Autodesk Inventor part; units mm, degrees
(part 2 of 2)
  line L623 (86.4105, 126.8852) -> (86.4105, 127.8852)
  line L624 (86.4105, 127.8852) -> (84.4105, 127.8852)
  line L625 (84.4105, 127.8852) -> (84.4105, 125.8852)
  line L626 (84.4105, 125.8852) -> (86.4105, 125.8852)
  line L627 (86.4105, 127.8852) -> (86.4105, 125.8852)
  line L628 (86.4105, 136.8852) -> (86.4105, 137.8852)
  line L629 (86.4105, 137.8852) -> (84.4105, 137.8852)
  line L630 (84.4105, 137.8852) -> (84.4105, 135.8852)
  line L631 (84.4105, 135.8852) -> (86.4105, 135.8852)
  line L632 (86.4105, 137.8852) -> (86.4105, 135.8852)
  line L633 (86.4105, 146.8852) -> (86.4105, 147.8852)
  line L634 (86.4105, 147.8852) -> (84.4105, 147.8852)
  line L635 (84.4105, 147.8852) -> (84.4105, 145.8852)
  line L636 (84.4105, 145.8852) -> (86.4105, 145.8852)
  line L637 (86.4105, 147.8852) -> (86.4105, 145.8852)
  line L638 (86.4105, 156.8852) -> (86.4105, 157.8852)
  line L639 (86.4105, 157.8852) -> (84.4105, 157.8852)
  line L640 (84.4105, 157.8852) -> (84.4105, 155.8852)
  line L641 (84.4105, 155.8852) -> (86.4105, 155.8852)
  line L642 (86.4105, 157.8852) -> (86.4105, 155.8852)
  line L643 (86.4105, 166.8852) -> (86.4105, 167.8852)
  line L644 (86.4105, 167.8852) -> (84.4105, 167.8852)
  line L645 (84.4105, 167.8852) -> (84.4105, 165.8852)
  line L646 (84.4105, 165.8852) -> (86.4105, 165.8852)
  line L647 (86.4105, 167.8852) -> (86.4105, 165.8852)
  line L648 (86.4105, 176.8852) -> (86.4105, 177.8852)
  line L649 (86.4105, 177.8852) -> (84.4105, 177.8852)
  line L650 (84.4105, 177.8852) -> (84.4105, 175.8852)
  line L651 (84.4105, 175.8852) -> (86.4105, 175.8852)
  line L652 (86.4105, 177.8852) -> (86.4105, 175.8852)
  line L653 (86.4105, 46.8852) -> (86.4105, 47.8852)
  line L654 (86.4105, 47.8852) -> (84.4105, 47.8852)
  line L655 (84.4105, 47.8852) -> (84.4105, 45.8852)
  line L656 (84.4105, 45.8852) -> (86.4105, 45.8852)
  line L657 (86.4105, 47.8852) -> (86.4105, 45.8852)
  line L658 (86.4105, 56.8852) -> (86.4105, 57.8852)
  line L659 (86.4105, 57.8852) -> (84.4105, 57.8852)
  line L660 (84.4105, 57.8852) -> (84.4105, 55.8852)
  line L661 (84.4105, 55.8852) -> (86.4105, 55.8852)
  line L662 (86.4105, 57.8852) -> (86.4105, 55.8852)
  line L663 (86.4105, 66.8852) -> (86.4105, 67.8852)
  line L664 (86.4105, 67.8852) -> (84.4105, 67.8852)
  line L665 (84.4105, 67.8852) -> (84.4105, 65.8852)
  line L666 (84.4105, 65.8852) -> (86.4105, 65.8852)
  line L667 (86.4105, 67.8852) -> (86.4105, 65.8852)
  line L668 (86.4105, 76.8852) -> (86.4105, 77.8852)
  line L669 (86.4105, 77.8852) -> (84.4105, 77.8852)
  line L670 (84.4105, 77.8852) -> (84.4105, 75.8852)
  line L671 (84.4105, 75.8852) -> (86.4105, 75.8852)
  line L672 (86.4105, 77.8852) -> (86.4105, 75.8852)
  line L673 (86.4105, 86.8852) -> (86.4105, 87.8852)
  line L674 (86.4105, 87.8852) -> (84.4105, 87.8852)
  line L675 (84.4105, 87.8852) -> (84.4105, 85.8852)
  line L676 (84.4105, 85.8852) -> (86.4105, 85.8852)
  line L677 (86.4105, 87.8852) -> (86.4105, 85.8852)
  line L678 (86.4105, 96.8852) -> (86.4105, 97.8852)
  line L679 (86.4105, 97.8852) -> (84.4105, 97.8852)
  line L680 (84.4105, 97.8852) -> (84.4105, 95.8852)
  line L681 (84.4105, 95.8852) -> (86.4105, 95.8852)
  line L682 (86.4105, 97.8852) -> (86.4105, 95.8852)
  line L683 (86.4105, 106.8852) -> (86.4105, 107.8852)
  line L684 (86.4105, 107.8852) -> (84.4105, 107.8852)
  line L685 (84.4105, 107.8852) -> (84.4105, 105.8852)
  line L686 (84.4105, 105.8852) -> (86.4105, 105.8852)
  line L687 (86.4105, 107.8852) -> (86.4105, 105.8852)
  line L688 (86.4105, 116.8852) -> (86.4105, 117.8852)
  line L689 (86.4105, 117.8852) -> (84.4105, 117.8852)
  line L690 (84.4105, 117.8852) -> (84.4105, 115.8852)
  line L691 (84.4105, 115.8852) -> (86.4105, 115.8852)
  line L692 (86.4105, 117.8852) -> (86.4105, 115.8852)
  line L693 (86.4105, 126.8852) -> (86.4105, 127.8852)
  line L694 (86.4105, 127.8852) -> (84.4105, 127.8852)
  line L695 (84.4105, 127.8852) -> (84.4105, 125.8852)
  line L696 (84.4105, 125.8852) -> (86.4105, 125.8852)
  line L697 (86.4105, 127.8852) -> (86.4105, 125.8852)
  line L698 (86.4105, 136.8852) -> (86.4105, 137.8852)
  line L699 (86.4105, 137.8852) -> (84.4105, 137.8852)
  line L700 (84.4105, 137.8852) -> (84.4105, 135.8852)
  line L701 (84.4105, 135.8852) -> (86.4105, 135.8852)
  line L702 (86.4105, 137.8852) -> (86.4105, 135.8852)
  line L703 (86.4105, 146.8852) -> (86.4105, 147.8852)
  line L704 (86.4105, 147.8852) -> (84.4105, 147.8852)
  line L705 (84.4105, 147.8852) -> (84.4105, 145.8852)
  line L706 (84.4105, 145.8852) -> (86.4105, 145.8852)
  line L707 (86.4105, 147.8852) -> (86.4105, 145.8852)
  line L708 (86.4105, 156.8852) -> (86.4105, 157.8852)
  line L709 (86.4105, 157.8852) -> (84.4105, 157.8852)
  line L710 (84.4105, 157.8852) -> (84.4105, 155.8852)
  line L711 (84.4105, 155.8852) -> (86.4105, 155.8852)
  line L712 (86.4105, 157.8852) -> (86.4105, 155.8852)
  line L713 (86.4105, 166.8852) -> (86.4105, 167.8852)
  line L714 (86.4105, 167.8852) -> (84.4105, 167.8852)
  line L715 (84.4105, 167.8852) -> (84.4105, 165.8852)
  line L716 (84.4105, 165.8852) -> (86.4105, 165.8852)
  line L717 (86.4105, 167.8852) -> (86.4105, 165.8852)
  line L718 (86.4105, 36.8852) -> (86.4105, 37.8852)
  line L719 (86.4105, 37.8852) -> (84.4105, 37.8852)
  line L720 (84.4105, 37.8852) -> (84.4105, 35.8852)
  line L721 (84.4105, 35.8852) -> (86.4105, 35.8852)
  line L722 (86.4105, 37.8852) -> (86.4105, 35.8852)
  line L723 (86.4105, 46.8852) -> (86.4105, 47.8852)
  line L724 (86.4105, 47.8852) -> (84.4105, 47.8852)
  line L725 (84.4105, 47.8852) -> (84.4105, 45.8852)
  line L726 (84.4105, 45.8852) -> (86.4105, 45.8852)
  line L727 (86.4105, 47.8852) -> (86.4105, 45.8852)
  line L728 (86.4105, 56.8852) -> (86.4105, 57.8852)
  line L729 (86.4105, 57.8852) -> (84.4105, 57.8852)
  line L730 (84.4105, 57.8852) -> (84.4105, 55.8852)
  line L731 (84.4105, 55.8852) -> (86.4105, 55.8852)
  line L732 (86.4105, 57.8852) -> (86.4105, 55.8852)
  line L733 (86.4105, 66.8852) -> (86.4105, 67.8852)
  line L734 (86.4105, 67.8852) -> (84.4105, 67.8852)
  line L735 (84.4105, 67.8852) -> (84.4105, 65.8852)
  line L736 (84.4105, 65.8852) -> (86.4105, 65.8852)
  line L737 (86.4105, 67.8852) -> (86.4105, 65.8852)
  line L738 (86.4105, 76.8852) -> (86.4105, 77.8852)
  line L739 (86.4105, 77.8852) -> (84.4105, 77.8852)
  line L740 (84.4105, 77.8852) -> (84.4105, 75.8852)
  line L741 (84.4105, 75.8852) -> (86.4105, 75.8852)
  line L742 (86.4105, 77.8852) -> (86.4105, 75.8852)
  line L743 (86.4105, 86.8852) -> (86.4105, 87.8852)
  line L744 (86.4105, 87.8852) -> (84.4105, 87.8852)
  line L745 (84.4105, 87.8852) -> (84.4105, 85.8852)
  line L746 (84.4105, 85.8852) -> (86.4105, 85.8852)
  line L747 (86.4105, 87.8852) -> (86.4105, 85.8852)
  line L748 (86.4105, 96.8852) -> (86.4105, 97.8852)
  line L749 (86.4105, 97.8852) -> (84.4105, 97.8852)
  line L750 (84.4105, 97.8852) -> (84.4105, 95.8852)
  line L751 (84.4105, 95.8852) -> (86.4105, 95.8852)
  line L752 (86.4105, 97.8852) -> (86.4105, 95.8852)
  line L753 (86.4105, 106.8852) -> (86.4105, 107.8852)
  line L754 (86.4105, 107.8852) -> (84.4105, 107.8852)
  line L755 (84.4105, 107.8852) -> (84.4105, 105.8852)
  line L756 (84.4105, 105.8852) -> (86.4105, 105.8852)
  line L757 (86.4105, 107.8852) -> (86.4105, 105.8852)
  line L758 (86.4105, 116.8852) -> (86.4105, 117.8852)
  line L759 (86.4105, 117.8852) -> (84.4105, 117.8852)
  line L760 (84.4105, 117.8852) -> (84.4105, 115.8852)
  line L761 (84.4105, 115.8852) -> (86.4105, 115.8852)
  line L762 (86.4105, 117.8852) -> (86.4105, 115.8852)
  line L763 (86.4105, 126.8852) -> (86.4105, 127.8852)
  line L764 (86.4105, 127.8852) -> (84.4105, 127.8852)
  line L765 (84.4105, 127.8852) -> (84.4105, 125.8852)
  line L766 (84.4105, 125.8852) -> (86.4105, 125.8852)
  line L767 (86.4105, 127.8852) -> (86.4105, 125.8852)
  line L768 (86.4105, 136.8852) -> (86.4105, 137.8852)
  line L769 (86.4105, 137.8852) -> (84.4105, 137.8852)
  line L770 (84.4105, 137.8852) -> (84.4105, 135.8852)
  line L771 (84.4105, 135.8852) -> (86.4105, 135.8852)
  line L772 (86.4105, 137.8852) -> (86.4105, 135.8852)
  line L773 (86.4105, 146.8852) -> (86.4105, 147.8852)
  line L774 (86.4105, 147.8852) -> (84.4105, 147.8852)
  line L775 (84.4105, 147.8852) -> (84.4105, 145.8852)
  line L776 (84.4105, 145.8852) -> (86.4105, 145.8852)
  line L777 (86.4105, 147.8852) -> (86.4105, 145.8852)
  line L778 (86.4105, 156.8852) -> (86.4105, 157.8852)
  line L779 (86.4105, 157.8852) -> (84.4105, 157.8852)
  line L780 (84.4105, 157.8852) -> (84.4105, 155.8852)
  line L781 (84.4105, 155.8852) -> (86.4105, 155.8852)
  line L782 (86.4105, 157.8852) -> (86.4105, 155.8852)
  line L783 (86.4105, 26.8852) -> (86.4105, 27.8852)
  line L784 (86.4105, 27.8852) -> (84.4105, 27.8852)
  line L785 (84.4105, 27.8852) -> (84.4105, 25.8852)
  line L786 (84.4105, 25.8852) -> (86.4105, 25.8852)
  line L787 (86.4105, 27.8852) -> (86.4105, 25.8852)
  line L788 (86.4105, 36.8852) -> (86.4105, 37.8852)
  line L789 (86.4105, 37.8852) -> (84.4105, 37.8852)
  line L790 (84.4105, 37.8852) -> (84.4105, 35.8852)
  line L791 (84.4105, 35.8852) -> (86.4105, 35.8852)
  line L792 (86.4105, 37.8852) -> (86.4105, 35.8852)
  line L793 (86.4105, 46.8852) -> (86.4105, 47.8852)
  line L794 (86.4105, 47.8852) -> (84.4105, 47.8852)
  line L795 (84.4105, 47.8852) -> (84.4105, 45.8852)
  line L796 (84.4105, 45.8852) -> (86.4105, 45.8852)
  line L797 (86.4105, 47.8852) -> (86.4105, 45.8852)
  line L798 (86.4105, 56.8852) -> (86.4105, 57.8852)
  line L799 (86.4105, 57.8852) -> (84.4105, 57.8852)
  line L800 (84.4105, 57.8852) -> (84.4105, 55.8852)
  line L801 (84.4105, 55.8852) -> (86.4105, 55.8852)
  line L802 (86.4105, 57.8852) -> (86.4105, 55.8852)
  line L803 (86.4105, 66.8852) -> (86.4105, 67.8852)
  line L804 (86.4105, 67.8852) -> (84.4105, 67.8852)
  line L805 (84.4105, 67.8852) -> (84.4105, 65.8852)
  line L806 (84.4105, 65.8852) -> (86.4105, 65.8852)
  line L807 (86.4105, 67.8852) -> (86.4105, 65.8852)
  line L808 (86.4105, 76.8852) -> (86.4105, 77.8852)
  line L809 (86.4105, 77.8852) -> (84.4105, 77.8852)
  line L810 (84.4105, 77.8852) -> (84.4105, 75.8852)
  line L811 (84.4105, 75.8852) -> (86.4105, 75.8852)
  line L812 (86.4105, 77.8852) -> (86.4105, 75.8852)
  line L813 (86.4105, 86.8852) -> (86.4105, 87.8852)
  line L814 (86.4105, 87.8852) -> (84.4105, 87.8852)
  line L815 (84.4105, 87.8852) -> (84.4105, 85.8852)
  line L816 (84.4105, 85.8852) -> (86.4105, 85.8852)
  line L817 (86.4105, 87.8852) -> (86.4105, 85.8852)
  line L818 (86.4105, 96.8852) -> (86.4105, 97.8852)
  line L819 (86.4105, 97.8852) -> (84.4105, 97.8852)
  line L820 (84.4105, 97.8852) -> (84.4105, 95.8852)
  line L821 (84.4105, 95.8852) -> (86.4105, 95.8852)
  line L822 (86.4105, 97.8852) -> (86.4105, 95.8852)
  line L823 (86.4105, 106.8852) -> (86.4105, 107.8852)
  line L824 (86.4105, 107.8852) -> (84.4105, 107.8852)
  line L825 (84.4105, 107.8852) -> (84.4105, 105.8852)
  line L826 (84.4105, 105.8852) -> (86.4105, 105.8852)
  line L827 (86.4105, 107.8852) -> (86.4105, 105.8852)
  line L828 (86.4105, 116.8852) -> (86.4105, 117.8852)
  line L829 (86.4105, 117.8852) -> (84.4105, 117.8852)
  line L830 (84.4105, 117.8852) -> (84.4105, 115.8852)
  line L831 (84.4105, 115.8852) -> (86.4105, 115.8852)
  line L832 (86.4105, 117.8852) -> (86.4105, 115.8852)
  line L833 (86.4105, 126.8852) -> (86.4105, 127.8852)
  line L834 (86.4105, 127.8852) -> (84.4105, 127.8852)
  line L835 (84.4105, 127.8852) -> (84.4105, 125.8852)
  line L836 (84.4105, 125.8852) -> (86.4105, 125.8852)
  line L837 (86.4105, 127.8852) -> (86.4105, 125.8852)
  line L838 (86.4105, 136.8852) -> (86.4105, 137.8852)
  line L839 (86.4105, 137.8852) -> (84.4105, 137.8852)
  line L840 (84.4105, 137.8852) -> (84.4105, 135.8852)
  line L841 (84.4105, 135.8852) -> (86.4105, 135.8852)
  line L842 (86.4105, 137.8852) -> (86.4105, 135.8852)
  line L843 (86.4105, 146.8852) -> (86.4105, 147.8852)
  line L844 (86.4105, 147.8852) -> (84.4105, 147.8852)
  line L845 (84.4105, 147.8852) -> (84.4105, 145.8852)
  line L846 (84.4105, 145.8852) -> (86.4105, 145.8852)
  line L847 (86.4105, 147.8852) -> (86.4105, 145.8852)
  point P0 (-17.2168, 0)
  dimension "d46" = 1
  dimension "d47" = 2
  dimension "d50" = 10
  dimension "d53" = 10
  constraints: 1692 end point, 840 vertical alignment, 504 collinear, 336 parallel, 4 perpendicular, 2 point on line, 1 midpoint, 1 vertical, 2 other
  measures "d46" distance of L3.start L3.end
  measures "d47" distance of L4.end L5.end
  measures "d50" distance of L3.start L8.start
  measures "d53" distance of L3.start L68.start
extrude "Выдавливание8" add sketch "Эскиз9" against normal blind 8 contours L0 L66 L2 L64 | L0 L61 L2 L59 | L54 L0 L56 L2 | L49 L0 L51 L2 | L44 L0 L46 L2 | L39 L0 L41 L2 | L34 L0 L36 L2 | L29 L0 L31 L2 | L24 L0 L26 L2 | L19 L0 L21 L2 | L14 L0 L16 L2 | L9 L0 L11 L2 | L4 L0 L6 L2 | L69 L0 L71 L2 | L134 L0 L136 L2 | L199 L0 L201 L2 | L264 L0 L266 L2 | L329 L0 L331 L2 | L394 L0 L396 L2 | L459 L0 L461 L2 | L524 L0 L526 L2 | L589 L0 L591 L2 | L654 L0 L656 L2 | L719 L0 L721 L2 | L784 L0 L786 L2
sketch "Эскиз10" plane through (128.3183, 0, 330) normal (1, 0, 0) x (0, 0, -1)
  point P0 (330, 0)
